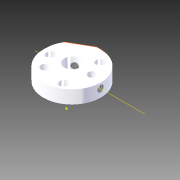
# Autodesk Inventor part: Tool Mount_Rev
Saved by Autodesk Inventor 2011 SP2 (Build 150309200, 309)
## iProperties
Created: 2011-04-05
Part Number: Tool Mount_Rev
Document SubType Name: Modeling
Designer: sungwook
Density: 1.42 g/cm^3
Material: Acetal Resin, White
Mass: 0.610937 g
Surface Area: 5.98911 cm^2
Volume: 0.430237 cm^3
Author: sungwook
Autodesk Inventor part; units mm, degrees
ref_plane "XZ Plane" through (0, 0, 0) normal (0, 1, 0) x (-1, 0, 0)
ref_plane "XY Plane" through (0, 0, 0) normal (0, 0, 1) x (1, 0, 0)
sketch "Sketch1" plane through (0, 0, 0) normal (0, 0, 1) x (1, 0, 0)
  circle A0 centre (1.5, 2.5981) radius 0.7125
  circle A1 centre (1.5, -2.5981) radius 0.7125
  circle A2 centre (-3, 0) radius 0.7125
  arc A3 (-7.6643, -2.2933) -> (-6.5192, -3.7417) centre (-5.2692, -1.5766) ccw
  line L0 (-6.5192, -3.7417) -> (0.0192, -7.5166)
  arc A4 (0.0192, -7.5166) -> (1.8461, -7.7841) centre (1.2692, -5.3516) ccw
  arc A5 (1.8461, -7.7841) -> (5.8182, -5.4908) centre (0, 0) ccw
  arc A6 (5.8182, -5.4908) -> (6.5, -3.7749) centre (4, -3.7749) ccw
  line L1 (6.5, -3.7749) -> (6.5, 3.7749)
  arc A7 (6.5, 3.7749) -> (5.8182, 5.4908) centre (4, 3.7749) ccw
  arc A8 (5.8182, 5.4908) -> (1.8461, 7.7841) centre (0, 0) ccw
  arc A9 (1.8461, 7.7841) -> (0.0192, 7.5166) centre (1.2692, 5.3516) ccw
  line L2 (0.0192, 7.5166) -> (-6.5192, 3.7417)
  arc A10 (-6.5192, 3.7417) -> (-7.6643, 2.2933) centre (-5.2692, 1.5766) ccw
  arc A11 (-7.6643, 2.2933) -> (-7.6643, -2.2933) centre (0, 0) ccw
  circle A12 centre (0, 0) radius 1.5
  circle A13 centre (-2, -3.4641) radius 0.25
  circle A14 centre (4, 0) radius 0.25
  circle A15 centre (-2, 3.4641) radius 0.25
  ellipse E0 centre (-6.667, 1.0078) end of major axis (-6.6776, 1.2132) minor radius 0.2
  ellipse E1 centre (2.4607, 6.2777) end of major axis (2.2881, 6.3896) minor radius 0.2
  ellipse E2 centre (2.4607, -6.2777) end of major axis (2.2881, -6.3896) minor radius 0.2
  ellipse E3 centre (-6.667, -1.0078) end of major axis (-6.6776, -1.2132) minor radius 0.2
  ellipse E4 centre (4.2063, 5.2699) end of major axis (4.3895, 5.1764) minor radius 0.2
  ellipse E5 centre (4.2063, -5.2699) end of major axis (4.3895, -5.1764) minor radius 0.2
  circle A16 centre (0, 0) radius 5.461
  circle A17 centre (0, 0) radius 4
  line L3 (-10.9328, 0) -> (9.5971, 0) projected
  line L4 (3.6555, 1.6239) -> (6.3662, 2.5383)
  line L5 (3.7085, -1.4989) -> (6.3662, -2.5383)
  point P0 (-4, 0)
  dimension "d0" = 10.922
  dimension "d1" = 8
  constraints: 21 point on circle, 18 centre point, 10 end point, 3 coincident, 2 point on line, 1 symmetric about line, 12 other
  measures "d0" diameter of A16
  measures "d1" diameter of A17
extrude "Extrusion1" add sketch "Sketch1" along normal blind 5.5 contours A0 | A1 | L3 A2 | L3 A12 A14 A17 A13 A2 | A2 L3 | A2 L3 A17 A15 A14 A12 | L3 A12 | A12 L3 | L3 A16 L4 A17 A15 | A17 A13 L5 A16 L3 | A17 A15 | A15 A17 | A17 A13 | A13 A17 | L3 A17 A14 | A14 A17 L3 | A16 L3 A14 A17 L4 | L5 A17 A14 L3 A16 | A14 L3 A17 | A17 L3 A14
hole "Hole1" [suppressed]
pattern_circular "Circular Pattern1" [suppressed]
extrude "Extrusion2" [suppressed]
sketch "Sketch2" plane through (0, 0, 5.5) normal (0, 0, 1) x (1, 0, 0)
  circle A0 centre (0, 0) radius 0.5 projected
  circle A1 centre (0, 0) radius 5.461 projected
  circle A2 centre (0, 0) radius 2
  circle A3 centre (0, 0) radius 1.6002
  dimension "d26" = 4
  dimension "d29" = 3.2004
  constraints: 2 centre point, 2 coincident
  measures "d26" diameter of A2
  measures "d29" diameter of A3
extrude "Extrusion4" [suppressed]
hole "Hole4" [suppressed]
sketch "Sketch4" plane through (0, 0, 0) normal (0, 0, -1) x (-1, 0, 0)
  circle A0 centre (0, 0) radius 5.461 projected
  circle A1 centre (0, 0) radius 1.85
  dimension "d52" = 3.7
  constraints: 1 centre point, 1 coincident
  measures "d52" diameter of A1
extrude "Extrusion6" cut sketch "Sketch4" against normal blind 2.5
hole "Hole5" [suppressed]
sketch "Sketch5" plane through (0, 0, 2.5) normal (0, 0, -1) x (-1, 0, 0)
  circle A0 centre (0, 0) radius 1.85 projected
  line L0 (-1.7812, 0.5) -> (-4, 0.5)
  line L1 (-4, 0.5) -> (-4, -0.5)
  line L2 (-4, -0.5) -> (-1.7812, -0.5)
  line L3 (-1.7812, -0.5) -> (-1.7812, 0.5)
  line L4 (7.6454, 0) -> (-7.6454, 0) projected
  point P0 (-4, 0)
  dimension "d64" = 1
  dimension "d65" = 4
  constraints: 8 end point, 2 parallel, 1 horizontal, 1 horizontal alignment, 1 midpoint, 1 perpendicular, 2 other
  measures "d64" distance between parallel lines of L2 L0
  measures "d65" distance from line of point (0, 0) L1
extrude "Extrusion7" [suppressed]
ref_plane "Work Plane1" through (5.461, 0, 0) normal (1, 0, 0) x (0, 1, 0)
sketch "Sketch6" plane through (5.461, 0, 0) normal (1, 0, 0) x (0, 1, 0)
  line L0 (-5.461, 5.5) -> (5.461, 5.5) projected
  line L1 (-5.461, 2.5) -> (-5.461, 5.5) projected
  line L2 (5.461, 2.5) -> (-5.461, 2.5) projected
  line L3 (5.461, 2.5) -> (5.461, 5.5) projected
  line L4 (0, -1.1) -> (0, 6.6) projected
  point P0 (0, 0)
  point P1 (0, 4)
  point P2 (0, 2.5)
  dimension "d110" = 3
  dimension "d111" = 1.5
  constraints: 2 point on line, 1 midpoint
  measures "d110" distance between parallel lines of L2 L0
  measures "d111" distance from line of L0 point (0, 4)
hole "Luer Attachment Hole" at (5.461, 0, 4) direction (-1, 0, 0) diameter 1.181 depth 5 thread size "0-80 UNF" class "2B" standard "ANSI Unified Screw Threads"
sketch "Sketch7" plane through (0, 0, 5.5) normal (0, 0, 1) x (1, 0, 0)
  circle A0 centre (0, 0) radius 5.461 projected
hole "Center Hole" at (0, 0, 5.5) direction (0, 0, -1) diameter 2.9972 end through all
pattern_circular "Circular Pattern2" count 2 over 120 about axis through (0, 0, -10) along (0, 0, 1) of "Luer Attachment Hole"
sketch "Sketch8" plane through (0, 0, 5.5) normal (0, 0, 1) x (1, 0, 0)
  circle A0 centre (0, 0) radius 5.461 projected
  circle A1 centre (0, 0) radius 3.9878
  line L0 (-7.7, 0) -> (7.7, 0) projected
  point P0 (-3.9878, 0)
  dimension "d87" = 7.9756
  constraints: 1 coincident, 1 horizontal alignment, 1 point on line, 2 other
hole "Hole8" at (-3.9878, 0, 5.5) direction (0, 0, -1) diameter 1.778 end through all countersink diameter 3.0226 countersink angle 82 clearance for "Flat Head Machine Screw (82)" size "#0" standard "Ansi Unified Screw Threads"
pattern_circular "Circular Pattern3" count 3 over 360 about axis through (0, 0, -10) along (0, 0, 1) of "Hole8"
chamfer "Chamfer1" [suppressed]
chamfer "Chamfer2" distance 0.5 angle 45 1 edges at (-2.7305, -4.7294, 5.5)
sketch "Sketch11" plane through (0, 0, 5.5) normal (0, 0, 1) x (1, 0, 0)
  circle A0 centre (0, 0) radius 1.4986 projected
  arc A1 (1.2893, 4.7905) -> (-4.7934, 1.2787) centre (0, 0) ccw projected
  arc A2 (-4.7934, -1.2787) -> (-4.7934, 1.2787) centre (-3.9878, 0) ccw projected
  arc A3 (-4.7934, -1.2787) -> (1.2893, -4.7905) centre (0, 0) ccw projected
  arc A4 (3.5041, -3.5118) -> (1.2893, -4.7905) centre (1.9939, -3.4535) ccw projected
  arc A5 (3.5041, -3.5118) -> (3.5041, 3.5118) centre (0, 0) ccw projected
  arc A6 (1.2893, 4.7905) -> (3.5041, 3.5118) centre (1.9939, 3.4535) ccw projected
  line L0 (0, 0) -> (-3.5779, 6.1972)
  line L1 (-7.7186, 0) -> (7.6589, 0) projected
  circle A7 centre (0, 0) radius 5.461 projected
  point P0 (-2.7305, 4.7294)
  dimension "d112" = 60
  constraints: 2 end point, 1 point on line, 2 other
  measures "d112" angle of L1 L0
ref_plane "Work Plane2" through (-2.7305, 4.7294, 5.5) normal (-0.5, 0.8660254, 0) x (-0.8660254, -0.5, 0)
sketch "Sketch12" plane through (-2.7305, 4.7294, 5.5) normal (-0.5, 0.8660254, 0) x (-0.8660254, -0.5, 0)
  arc A0 (-3.5118, 0) -> (-4.7905, 0) centre (-4.7905, 0) ccw projected
  line L0 (-4.7905, 0) -> (-1.2787, 0) projected
  arc A1 (-1.2787, 0) -> (1.2787, 0) centre (1.2787, 0) ccw projected
  line L1 (1.2787, 0) -> (4.7905, 0) projected
  arc A2 (4.7905, 0) -> (3.5118, 0) centre (3.5118, 0) ccw projected
  line L2 (3.5118, 0) -> (-3.5118, 0) projected
  line L3 (5.461, -0.5) -> (-5.461, -0.5) projected
  line L4 (5.461, -0.5) -> (-5.461, -0.5) projected
  line L5 (13.0759, -1.5) -> (-12.0496, -1.5) projected
  line L6 (0, -6.6212) -> (0, 1.227) projected
  line L7 (-5.461, -3) -> (-5.461, -0.5) projected
  line L8 (5.461, -3) -> (5.461, -0.5) projected
  line L9 (5.461, -3) -> (-5.461, -3) projected
  line L10 (-5.461, -3) -> (5.461, -3)
  line L11 (5.461, -3) -> (5.461, 0)
  line L12 (5.461, 0) -> (-5.461, 0)
  line L13 (-5.461, 0) -> (-5.461, -3)
  point P0 (0, -5.5)
  constraints: 8 end point, 3 horizontal alignment, 2 parallel, 1 horizontal, 1 perpendicular, 1 point on line
extrude "Extrusion8" cut sketch "Sketch12" against normal blind 1 contours L0 A1 L3 L13 L12 | L2 L6 L3 A1 | L3 A1 L5 L7 | L3 L6 L5 A1 | L2 A1 L3 L6 | L5 A1 L9 L7 | L5 L6 L9 A1 | L3 A1 L5 L6 | L1 L12 L11 L3 A1 | L5 A1 L9 L6 | L3 L8 L5 A1 | L5 L8 L9 A1
sketch "Sketch16" plane through (0, 0, 5.5) normal (0, 0, 1) x (1, 0, 0)
  arc A0 (-4.1102, 2.7781) -> (-4.7934, 1.2787) centre (0, 0) ccw projected
  line L0 (-7.7186, 0) -> (7.6589, 0) projected
  point P0 (3.81, 0)
  point P1 (-1.905, 3.2996)
  point P2 (-1.905, -3.2996)
  dimension "d117" = 3.81
  dimension "d120" = 360
  constraints: 1 point on line, 4 other
  measures "d117" distance of point (3.81, 0) A0.centre
hole "Hole9" at (3.81, 0, 5.5) at (-1.905, -3.2996, 5.5) direction (0, 0, -1) diameter 1.4732 end through all
sketch "Sketch17" plane through (-2.2305, 3.8633, 5.5) normal (-0.5, 0.8660254, 0) x (0.8660254, 0.5, 0)
  arc A0 (3.1499, 0.5) -> (2.1705, 0) centre (2.1705, 0) ccw projected
  line L0 (3.1499, 3) -> (3.1499, 0.5) projected
  line L1 (-3.1499, 3) -> (3.1499, 3) projected
  line L2 (-3.1499, 0.5) -> (-3.1499, 3) projected
  arc A1 (-2.1705, 0) -> (-3.1499, 0.5) centre (-3.1499, 0.5) ccw projected
  line L3 (2.1705, 0) -> (-2.1705, 0) projected
  circle A2 centre (0, 1.5) radius 0.5905 projected
  point P0 (0, 5.5)
  constraints: 2 other
ref_plane "Work Plane3" through (-2.2305, 3.8633, 4) normal (-0.5, 0.8660254, 0) x (0.8660254, 0.5, 0)
equation "\"d111\" = 0.5 * d110"
equation "\"d68\" = 0.5 * d0"
body "Solid1"
